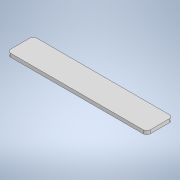
# Autodesk Inventor part: верхняя защелка башни
Saved by Autodesk Inventor 2020.1 (Build 241239000, 239)
## iProperties
Created: 2022-04-03
Part Number: верхняя защелка башни
Material: Типовые
Document SubType Name: Modeling
Designer: User
Density: 1 g/cm^3
Appearance: По умолчанию
Author: User
Autodesk Inventor part; units mm, degrees
ref_plane "YZ Plane" through (0, 0, 0) normal (1, 0, 0) x (0, 1, 0)
ref_plane "XZ Plane" through (0, 0, 0) normal (0, 1, 0) x (-1, 0, 0)
ref_plane "XY Plane" through (0, 0, 0) normal (0, 0, 1) x (1, 0, 0)
sketch "Эскиз1" plane through (0, 0, 0) normal (0, 1, 0) x (-1, 0, 0)
  line L0 (0, 0) -> (-15, 0)
  line L1 (-15, 0) -> (-15, -5)
  line L2 (-15, -5) -> (0, -5)
  line L3 (0, -5) -> (0, 0)
  dimension "d0" = 5
  dimension "d1" = 15
  constraints: 8 end point, 2 parallel, 1 horizontal, 1 perpendicular
  measures "d0" distance of L2.end L0.start
  measures "d1" distance of L1.end L2.end
extrude "Выдавливание1" add sketch "Эскиз1" along normal blind 4
sketch "Эскиз2" plane through (0, 4, 0) normal (0, 1, 0) x (1, 0, 0)
  line L0 (-10, -5) -> (30, -5)
  line L1 (30, -5) -> (30, 10)
  line L2 (30, 10) -> (-10, 10)
  line L3 (-10, 10) -> (-10, -5)
  line L4 (-10, 2.5) -> (-4.0843, 2.5)
  line L5 (0, 5) -> (0, 0) projected
  line L6 (0, 2.5) -> (15, 2.5)
  line L7 (15, 0) -> (15, 5) projected
  dimension "d4" = 10
  dimension "d5" = 5
  dimension "d6" = 15
  constraints: 12 end point, 3 midpoint, 2 horizontal, 2 parallel, 1 perpendicular, 1 other
  measures "d4" distance between parallel lines of L5 L3
  measures "d5" distance from line of L2 L7.end
  measures "d6" distance from line of L1 L7.end
extrude "Выдавливание2" add sketch "Эскиз2" along normal blind 2
fillet "Сопряжение1" radius 2 2 edges at (30, 5, 5) (30, 5, -10)
mirror "Зеркальное отражение1" about plane through (-10, 4, -10) normal (-1, 0, 0)
